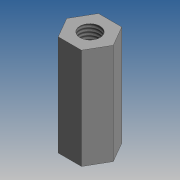
# Autodesk Inventor part: P043_entretoise15par3
Saved by Autodesk Inventor 2021.3 (Build 253353000, 353)
## iProperties
Created: 2021-12-17
Part Number: P043_entretoise15par3
Material: Générique
Document SubType Name: Modeling
Designer: gabri
Density: 1 g/cm^3
Appearance: Par défaut
Author: gabri
Autodesk Inventor part; units mm, degrees
ref_plane "YZ Plane" through (0, 0, 0) normal (1, 0, 0) x (0, 1, 0)
ref_plane "XZ Plane" through (0, 0, 0) normal (0, 1, 0) x (-1, 0, 0)
ref_plane "XY Plane" through (0, 0, 0) normal (0, 0, 1) x (1, 0, 0)
sketch "Sketch2" plane through (0, 0, 0) normal (0, 0, 1) x (1, 0, 0)
  line L0 (-1.7321, 3) -> (1.7321, 3)
  line L1 (1.7321, 3) -> (3.4641, 0)
  line L2 (3.4641, 0) -> (1.7321, -3)
  line L3 (1.7321, -3) -> (-1.7321, -3)
  line L4 (-1.7321, -3) -> (-3.4641, 0)
  line L5 (-3.4641, 0) -> (-1.7321, 3)
  line L6 (-4.8497, 0) -> (4.8497, 0) construction
  circle A0 centre (0, 0) radius 1.5
  dimension "d0" = 6
  dimension "d3" = 3
  constraints: 12 end point, 2 coincident, 1 centre point, 1 parallel, 13 other
  measures "d0" distance between parallel lines of L3 L0
  measures "d3" diameter of A0
extrude "Extrusion1" add sketch "Sketch2" along normal blind 15
thread "Thread1" size "M3x0.5" class "6H" standard "ISO Metric profile" full length
body "Solid1"
